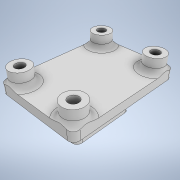
# Autodesk Inventor part: turbidity-pcb-mount
Saved by Autodesk Inventor 2020.1 (Build 241239000, 239)
## iProperties
Created: 2019-11-14
Part Number: turbidity-pcb-mount
Material: Generic
Document SubType Name: Modeling
Designer: njk024
Density: 1 g/cm^3
Appearance: Default
Author: njk024
Autodesk Inventor part; units mm, degrees
ref_plane "YZ Plane" through (0, 0, 0) normal (1, 0, 0) x (0, 1, 0)
ref_plane "XZ Plane" through (0, 0, 0) normal (0, 1, 0) x (-1, 0, 0)
ref_plane "XY Plane" through (0, 0, 0) normal (0, 0, 1) x (1, 0, 0)
sketch "Sketch1" plane through (0, 0, 0) normal (0, 1, 0) x (-1, 0, 0)
  circle A0 centre (0, 0) radius 1.65
  circle A1 centre (0, -30) radius 1.65
  circle A2 centre (-20, 0) radius 1.65
  circle A3 centre (-20, -30) radius 1.65
  line L0 (0, 0) -> (-20, 0) construction
  line L1 (-20, 0) -> (-20, -30) construction
  line L2 (-20, -30) -> (0, -30) construction
  line L3 (0, -30) -> (0, 0) construction
  line L4 (4, 4) -> (-24, 4)
  line L5 (-24, 4) -> (-24, -34)
  line L6 (-24, -34) -> (4, -34)
  line L7 (4, -34) -> (4, 4)
  dimension "d1" = 3.3
  dimension "d2" = 3.3
  dimension "d4" = 3.3
  dimension "d5" = 3.3
  dimension "d6" = 30
  dimension "d7" = 20
  dimension "d8" = 4
  constraints: 16 end point, 4 centre point, 4 parallel, 3 coincident, 2 perpendicular, 1 horizontal, 3 other
  measures "d1" diameter of A0
  measures "d2" diameter of A1
  measures "d4" diameter of A2
  measures "d5" diameter of A3
  measures "d6" distance of L2.end L0.start
  measures "d7" distance of L0.start L0.end
  measures "d8" distance between parallel lines of L4 L0
extrude "Extrusion1" add sketch "Sketch1" along normal blind 3
sketch "Sketch2" plane through (0, 0, 0) normal (0, -1, 0) x (1, 0, 0)
  circle A0 centre (20, -30) radius 1.65 construction
  circle A1 centre (20, 0) radius 1.65 construction
  circle A2 centre (0, -30) radius 1.65 construction
  circle A3 centre (0, 0) radius 1.65 construction
  line L0 (24, -34) -> (-4, -34) projected
  line L1 (-4, -34) -> (-4, 4) projected
  line L2 (-4, 4) -> (24, 4) projected
  line L3 (24, 4) -> (24, -34) projected
  line L4 (16, -26) -> (4, -26)
  line L5 (4, -26) -> (4, -4)
  line L6 (4, -4) -> (16, -4)
  line L7 (16, -4) -> (16, -26)
  dimension "d11" = 8
  constraints: 8 end point, 3 other
  measures "d11" distance between parallel lines of L3 L7
extrude "Extrusion2" add sketch "Sketch2" along normal blind 12 contours L4 L5 L6 L7
fillet "Fillet1" radius 2 8 edges at (24, 1.5, 4) (-4, 1.5, 4) (-4, 1.5, -34) (24, 1.5, -34) (16, -6, -4) (4, -6, -4) (4, -6, -26) (16, -6, -26)
sketch "Sketch3" plane through (0, 3, 0) normal (0, 1, 0) x (1, 0, 0)
  circle A0 centre (0, 0) radius 1.65 projected
  circle A1 centre (0, 30) radius 1.65 projected
  circle A2 centre (20, 0) radius 1.65 projected
  circle A3 centre (20, 30) radius 1.65 projected
  circle A4 centre (0, 0) radius 3.5
  circle A5 centre (0, 30) radius 1.65 projected
  circle A6 centre (0, 30) radius 3.5
  circle A7 centre (20, 0) radius 1.65 projected
  circle A8 centre (20, 0) radius 3.5
  circle A9 centre (20, 30) radius 3.5
  dimension "d15" = 7
  dimension "d16" = 7
  dimension "d17" = 7
  dimension "d18" = 7
  constraints: 4 centre point, 4 coincident
  measures "d15" diameter of A4
  measures "d16" diameter of A6
  measures "d17" diameter of A8
  measures "d18" diameter of A9
extrude "Extrusion3" add sketch "Sketch3" along normal blind 5
fillet "Fillet2" radius 2 4 edges at (-3.5, 3, 0) (-3.5, 3, -30) (16.5, 3, 0) (16.5, 3, -30)
body "Solid1"
